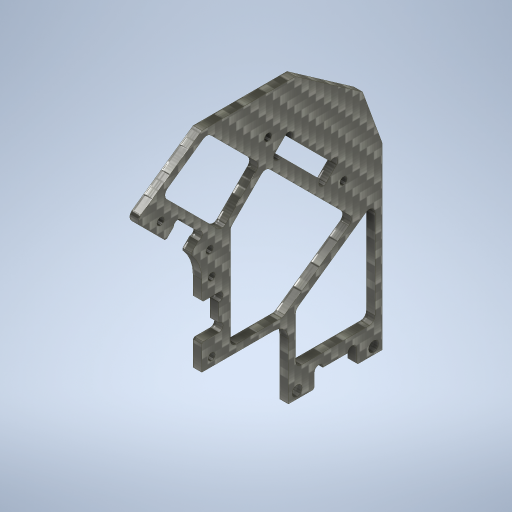
# Autodesk Inventor part: HeadSideFrame
Saved by Autodesk Inventor 2024.2 (Build 282272000, 272)
## iProperties
Created: 2024-01-28
Part Number: HeadSideFrame
Material: CFRP
Document SubType Name: Modeling
Designer: Masato Kubotera
Density: 1.43 g/cm^3
Appearance: Carbon Fiber 1
Mass: 10.5129 g
Surface Area: 73.9298 cm^2
Volume: 7.35165 cm^3
Vendor: meviy
Author: Masato Kubotera
Autodesk Inventor part; units mm, degrees
ref_plane "YZ Plane" through (0, 0, 0) normal (1, 0, 0) x (0, 1, 0)
ref_plane "XY Plane" through (0, 0, 0) normal (0, 0, 1) x (1, 0, 0)
ref_plane "Work Plane1" through (0, 30, 0) normal (0, 1, 0) x (-1, 0, 0)
sketch "Sketch1" plane through (0, 30, 0) normal (0, 1, 0) x (-1, 0, 0)
  line L0 (-16.25, -1.5) -> (16.25, -1.5)
  line L1 (-7.3, -1.5) -> (-7.3, 3.5)
  line L2 (7.3, 3.5) -> (7.3, -1.5)
  arc A0 (7.3, 3.5) -> (4.3, 3.5) centre (5.8, 3.5) ccw
  arc A1 (-4.3, 3.5) -> (-7.3, 3.5) centre (-5.8, 3.5) ccw
  line L3 (0, -1.5) -> (0, 3.5) construction
  line L4 (-13.25, 1) -> (13.25, 1) construction
  line L5 (-7.25, -1.5) -> (-7.25, 3.5) construction
  line L6 (7.25, -1.5) -> (7.25, 3.5) construction
  arc A2 (-47.5142, 62.9298) -> (-47.5142, 65.9298) centre (-47.5142, 64.4298) ccw
  line L7 (-62.6665, 77.5467) -> (-41.4533, 56.3335) construction
  line L8 (-33.1802, 64.6066) -> (-54.3934, 85.8198) construction
  line L9 (-53.8277, 65.1723) -> (-50.2922, 68.7078) construction
  arc A3 (-53.0702, 71.4858) -> (-56.0702, 71.4858) centre (-54.5702, 71.4858) ccw
  line L10 (-49.5851, 60.9296) -> (-46.0495, 64.4652) construction
  line L11 (-54.5348, 72.9505) -> (-49.5851, 60.9296) construction
  line L12 (-46.0495, 64.4652) -> (-54.5348, 72.9505) construction
  line L13 (-46.0495, 64.4652) -> (-58.0704, 69.4149) construction
  line L14 (-54.5348, 72.9505) -> (-58.0704, 69.4149) construction
  line L15 (-58.0704, 69.4149) -> (-49.5851, 60.9296) construction
  line L16 (-54.5702, 72.9858) -> (-58.7421, 68.8139)
  line L17 (-62.7373, 44.2419) -> (-46.0495, 60.9296) construction
  line L18 (-41.4533, 56.3335) -> (-33.1802, 64.6066) construction
  line L19 (-46.0142, 64.4298) -> (-54.5702, 72.9858)
  line L20 (-60.5452, 75.4253) -> (-43.5747, 58.4548) construction
  line L21 (-74.7581, 56.2627) -> (-62.7373, 44.2419) construction
  line L22 (-58.0704, 72.9505) -> (-74.7581, 56.2627) construction
  line L23 (-54.3934, 85.8198) -> (-62.6665, 77.5467) construction
  line L24 (-65, 54) -> (-119, 0) construction
  line L25 (0, 0) -> (-119, 0) construction
  line L26 (2.5776, 98) -> (57.5979, 98) construction
  line L27 (-7.3, 3.5) -> (7.3, 3.5)
  line L28 (-46.25, 98) -> (-46.25, 23) construction
  ellipse E0 centre (-46.25, 60.5) end of major axis (-46.25, 98) minor radius 30 (-46.25, 98) -> (-46.25, 23) ccw construction
  line L29 (-30, 98) -> (-30, 23) construction
  ellipse E1 centre (-13.75, 60.5) end of major axis (-13.75, 98) minor radius 30 (-13.75, 23) -> (-13.75, 98) ccw construction
  line L30 (-46.25, 98) -> (-13.75, 98) construction
  line L31 (-46.25, 23) -> (-13.75, 23) construction
  line L32 (-58.9896, 47.9896) -> (-71.0104, 60.0104) construction
  line L33 (-57.5883, 31.2154) -> (-87.7846, 61.4117) construction
  line L34 (-65, 54) -> (-57.5883, 31.2154) construction
  line L35 (-65, 54) -> (-87.7846, 61.4117) construction
  line L36 (-46.0142, 64.4298) -> (-50.1861, 60.2579)
  line L37 (-58.7421, 68.8139) -> (-69.2932, 79.365)
  line L38 (16.25, -1.5) -> (16.25, 60.5)
  line L39 (-16.25, -1.5) -> (-16.25, 23)
  line L40 (-20.8731, 76.0546) -> (-17.3376, 79.5901) construction
  line L41 (-17.3376, 79.5901) -> (0.3401, 61.9124) construction
  line L42 (0.3401, 61.9124) -> (-3.1954, 58.3769) construction
  line L43 (-3.1954, 58.3769) -> (-20.8731, 76.0546) construction
  line L44 (-20.8731, 76.0546) -> (0.3401, 61.9124) construction
  line L45 (-17.3376, 79.5901) -> (-3.1954, 58.3769) construction
  line L46 (-20.9438, 76.0546) -> (-17.3376, 79.6608)
  line L47 (-17.3376, 79.6608) -> (0.4108, 61.9124)
  line L48 (0.4108, 61.9124) -> (-3.1954, 58.3062)
  line L49 (-3.1954, 58.3062) -> (-20.9438, 76.0546)
  line L50 (-20.9438, 76.0546) -> (0.4108, 61.9124) construction
  line L51 (-17.3376, 79.6608) -> (-3.1954, 58.3062) construction
  arc A4 (-15.2163, 77.5395) -> (-17.3376, 79.6608) centre (-16.2769, 78.6001) ccw
  line L52 (-35.0152, 93.7322) -> (14.4822, 44.2348) construction
  line L53 (-8.4634, 70.7866) -> (-12.0696, 67.1804) construction
  arc A5 (-20.9438, 76.0546) -> (-18.8225, 73.9332) centre (-19.8832, 74.9939) ccw
  arc A6 (0.4108, 61.9124) -> (-1.7105, 64.0337) centre (-0.6499, 62.9731) ccw
  arc A7 (-5.3168, 60.4275) -> (-3.1954, 58.3062) centre (-4.2561, 59.3668) ccw
  line L54 (-46.25, 50.7553) -> (-46.25, 23)
  line L55 (-33.2475, 95.5) -> (-36.783, 91.9645) construction
  line L56 (-40.35, 32) -> (-46.25, 32) construction
  line L57 (-46.25, 44) -> (-40.35, 44) construction
  line L58 (-40.35, 44) -> (-40.35, 32) construction
  line L59 (-40.35, 32) -> (-46.25, 44) construction
  line L60 (-46.25, 32) -> (-40.35, 44) construction
  line L61 (-46.25, 44.05) -> (-40.35, 44.05)
  line L62 (-40.35, 44.05) -> (-40.35, 31.95)
  line L63 (-40.35, 31.95) -> (-46.25, 31.95)
  line L64 (-40.35, 38) -> (-46.25, 38) construction
  arc A8 (-40.35, 41.05) -> (-40.35, 44.05) centre (-40.35, 42.55) ccw
  line L65 (-42.85, 50) -> (-42.85, 26) construction
  line L66 (-46.25, 53) -> (-40.35, 53) construction
  arc A9 (-40.35, 31.95) -> (-40.35, 34.95) centre (-40.35, 33.45) ccw
  line L67 (-65.0707, 75.1425) -> (-60.8988, 79.3144) construction
  line L68 (-43.2211, 54.5657) -> (-39.6856, 58.1012) construction
  line L69 (-46.25, 60.5) -> (-76.25, 60.5) construction
  line L70 (-13.75, 60.5) -> (16.25, 60.5) construction
  line L71 (-11.75, 8) -> (11.75, 8)
  line L72 (-46.25, 95.5) -> (-13.75, 95.5)
  line L73 (-50.1861, 60.2579) -> (-46.25, 64.194)
  circle A10 centre (-42.85, 26) radius 2.4 construction
  circle A11 centre (-60.5452, 75.4253) radius 2.4 construction
  line L74 (-50.1861, 60.2579) -> (-50.1861, 60.2579)
  line L75 (4.9456, 44.5083) -> (-22.7522, 72.2061)
  line L76 (-25.5807, 72.2061) -> (-35.7642, 62.0226)
  line L77 (-36.35, 60.6084) -> (-36.35, 27.5)
  line L78 (-27.3484, 76.8023) -> (-43.1484, 92.6023)
  line L79 (-27.3484, 73.9739) -> (-37.9607, 63.3616)
  line L80 (-40.7891, 63.3616) -> (-58.4603, 81.0328)
  line L81 (-18.7392, 25.5) -> (-34.35, 25.5)
  line L82 (9.4147, 79.2799) -> (16.25, 60.5)
  line L83 (-13.75, 98) -> (-13.75, 23) construction
  line L84 (-13.75, 95.5) -> (9.4147, 79.2799)
  line L85 (16.25, 60.5) -> (9.4147, 41.7201)
  line L86 (9.4147, 41.7201) -> (-12.8972, 26.0972)
  line L87 (-46.25, 23) -> (-16.25, 23)
  line L88 (-13.75, 24.4589) -> (-13.75, 10)
  line L89 (13.75, 10) -> (13.75, 40.9137)
  line L90 (-46.25, 95.5) -> (-69.2932, 79.365)
  line L91 (9.4147, 41.7201) -> (10.6028, 42.552)
  line L92 (4.6786, 41.4558) -> (-17.5921, 25.8617)
  line L93 (-58.1932, 84.0853) -> (-45.7097, 92.8264)
  arc A12 (-43.1484, 92.6023) -> (-45.7097, 92.8264) centre (-44.5626, 91.1881) ccw
  arc A13 (-58.1932, 84.0853) -> (-58.4603, 81.0328) centre (-57.0461, 82.447) ccw
  arc A14 (-40.7891, 63.3616) -> (-37.9607, 63.3616) centre (-39.3749, 64.7758) ccw
  arc A15 (-27.3484, 73.9739) -> (-27.3484, 76.8023) centre (-28.7626, 75.3881) ccw
  arc A16 (-22.7522, 72.2061) -> (-25.5807, 72.2061) centre (-24.1665, 70.7919) ccw
  arc A17 (4.6786, 41.4558) -> (4.9456, 44.5083) centre (3.5314, 43.0941) ccw
  arc A18 (-18.7392, 25.5) -> (-17.5921, 25.8617) centre (-18.7392, 27.5) ccw
  arc A19 (-36.35, 27.5) -> (-34.35, 25.5) centre (-34.35, 27.5) ccw
  arc A20 (-35.7642, 62.0226) -> (-36.35, 60.6084) centre (-34.35, 60.6084) ccw
  arc A21 (13.75, 40.9137) -> (10.6028, 42.552) centre (11.75, 40.9137) ccw
  arc A22 (-12.8972, 26.0972) -> (-13.75, 24.4589) centre (-11.75, 24.4589) ccw
  arc A23 (-13.75, 10) -> (-11.75, 8) centre (-11.75, 10) ccw
  arc A24 (11.75, 8) -> (13.75, 10) centre (11.75, 10) ccw
  arc A25 (-46.25, 50.7553) -> (-50.1861, 60.2579) centre (-59.6887, 50.7553) ccw
  line L94 (12.7145, 42.467) -> (16.25, 46.0025) construction
  point P0 (-52.0599, 66.9401)
  point P1 (-47.5142, 65.9298)
  point P2 (-72.6865, 46.3135)
  point P3 (-76.1621, 57.6309)
  point P4 (-74.597, 48.2241)
  point P5 (-46.0142, 64.4298)
  point P6 (-46.0142, 64.4298)
  point P7 (-16.25, 34)
  point P8 (-10.2665, 68.9835)
  point P9 (-46.25, 56.3218)
  point P10 (-23.348, 82.065)
  point P11 (2.815, 55.902)
  point P12 (-1.7105, 64.0337)
  point P13 (-5.3168, 60.4275)
  point P14 (-18.8225, 73.9332)
  point P15 (-43.3, 38)
  point P16 (-40.35, 34.95)
  point P17 (-73.75, 60.5)
  point P18 (-13.75, 8)
  point P19 (13.75, 8)
  point P20 (16.25, 71.5)
  point P21 (-40.35, 45.95)
  point P22 (-47.0041, 71.6114)
  point P23 (6.631, 42.8229)
  point P24 (-24.1665, 73.6203)
  point P25 (-36.35, 61.4368)
  point P26 (-36.35, 25.5)
  point P27 (-25.9342, 75.3881)
  point P28 (-44.335, 93.7889)
  point P29 (-71.25, 60.5)
  point P30 (-39.3749, 61.9474)
  point P31 (-60.1457, 82.7182)
  point P32 (-13.75, 25.5)
  point P33 (13.75, 53.6313)
  point P34 (13.75, 44.7557)
  point P35 (-18.1086, 25.5)
  point P36 (-50.1861, 60.2579)
  dimension "d26" = 30
  dimension "d1" = 32.5
  dimension "d2" = 1.5
  dimension "d3" = 1.5
  dimension "d4" = 0.05
  dimension "d5" = 6
  dimension "d6" = 11.7
  dimension "d7" = 35.3
  dimension "d8" = 30
  dimension "d9" = 17
  dimension "d10" = 30
  dimension "d11" = 0.05
  dimension "d12" = 5
  dimension "d14" = 6
  dimension "d15" = 45
  dimension "d16" = 65
  dimension "d17" = 54
  dimension "d18" = 98
  dimension "d19" = 1.5
  dimension "d20" = 2.5
  dimension "d22" = 5
  dimension "d24" = 75
  dimension "d25" = 30
  dimension "d32" = 76.3675
  dimension "d34" = 10.8703
  dimension "d35" = 21.352
  dimension "d44" = 32.5
  dimension "d50" = 9
  dimension "d55" = 5
  dimension "d56" = 25
  dimension "d60" = 6
  dimension "d61" = 0.05
  dimension "d62" = 0.05
  dimension "d64" = 0.05
  dimension "d67" = 5.9
  dimension "d68" = 6
  dimension "d70" = 9
  dimension "d71" = 9
  dimension "d75" = 2.5
  dimension "d76" = 30
  dimension "d81" = 3
  dimension "d96" = 4.8
  dimension "d97" = 0.6
  dimension "d98" = 15
  dimension "d99" = 2.5
  dimension "d100" = 1
  dimension "d101" = 1
  dimension "d103" = 2.5
  dimension "d104" = 2.5
  dimension "d106" = 2.5
  dimension "d108" = 2.5
  dimension "d109" = 145
  dimension "d110" = 145
  dimension "d111" = 2.5
  dimension "d112" = 140
  dimension "d113" = 2
  dimension "d117" = 2.5
  dimension "d118" = 2.5
  dimension "d119" = 2.5
  dimension "d120" = 70
  dimension "d121" = 45
  dimension "d122" = 30
  constraints: 192 end point, 76 point on line, 49 point on circle, 28 tangent, 26 centre point, 24 midpoint, 23 symmetric about line, 16 equal radius, 16 parallel, 15 perpendicular, 14 horizontal, 12 collinear, 9 coincident, 8 vertical, 27 other
  measures "d1" distance of L0.start L0.end
  measures "d2" radius of A0
  measures "d3" distance from line of L0 L25.start
  measures "d4" distance between parallel lines of L2 L6
  measures "d5" distance from line of point (13.25, 1) L6
  measures "d6" distance of L7.end L8.start
  measures "d7" distance between parallel lines of L21 L8
  measures "d8" distance from line of L34.start L8
  measures "d9" distance between parallel lines of L17 L22
  measures "d10" distance of L8.start L8.end
  measures "d11" distance between parallel lines of L16 L14
  measures "d12" distance between parallel lines of L15 L12
  measures "d14" distance from line of L20.start L14
  measures "d15" angle of L24 L3
  measures "d16" horizontal distance of L25.start L34.start
  measures "d17" vertical distance of L25.start L34.start
  measures "d18" distance from line of L25.start L26
  measures "d19" radius of A3
  measures "d20" distance between parallel lines of L12 L7
  measures "d22" distance between parallel lines of L0 L27
  measures "d24" distance of L28.start L31.start
  measures "d25" distance from line of L25.start L29
  measures "d32" distance of L34.start L25.end
  measures "d34" distance from line of L33 L34.start
  measures "d35" distance of point (-72.686, 46.314) L33.end
  measures "d44" distance of L31.start L31.end
  measures "d50" distance from line of L0.end L6
  measures "d55" distance of L40.start L40.end
  measures "d56" distance of L40.end L41.end
  measures "d60" distance from line of L40 point (-23.348, 82.065)
  measures "d61" distance between parallel lines of L46 L40
  measures "d62" distance between parallel lines of L41 L47
  measures "d64" distance between parallel lines of L57 L61
  measures "d67" distance of L61.start L61.end
  measures "d68" distance from line of L57 L65.start
  measures "d70" distance between parallel lines of L57 L66
  measures "d71" distance between parallel lines of L67 L14
  measures "d75" distance of L69.end point (-73.75, 60.5)
  measures "d76" diameter of L66 L64
  measures "d81" distance edge to line of A0 L71
  measures "d96" diameter of A10
  measures "d97" distance edge to line of A10 L31
  measures "d98" distance between parallel lines of L31 L64
  measures "d99" distance between parallel lines of L62 L65
  measures "d100" distance edge to line of A10 L54
  measures "d101" distance edge to line of A11 L37
  measures "d103" distance edge to line of A9 L77
  measures "d104" distance edge to line of A7 L75
  measures "d106" distance of point (-73.75, 60.5) point (-71.25, 60.5)
  measures "d108" distance between parallel lines of L79 L76
  measures "d109" angle of L82 L84
  measures "d110" angle of L84 L72
  measures "d111" distance between parallel lines of L72 L30
  measures "d112" angle of L85 L82
  measures "d113" radius of A12
  measures "d117" distance between parallel lines of L86 L92
  measures "d118" distance between parallel lines of L90 L93
  measures "d119" distance edge to line of A2 L80
  measures "d120" distance between parallel lines of L94 L55
  measures "d121" angle of L29 L52
  measures "d122" distance between parallel lines of L68 L67
extrude "Extrusion1" add sketch "Sketch1" against normal blind 3 contours L39 L87 L54 L63 A9 L62 A8 L61 A25 L36 A2 L19 A3 L16 L37 L90 L72 L84 L82 L38 L0 L2 A0 L27 A1 L1
hole "Hole1" at (13.25, 30, 1) at (-13.25, 30, 1) direction (0, -1, 0) diameter 3.5 end through all
hole "Hole2" at (60.5452, 30, 75.4253) at (43.5747, 30, 58.4548) at (65, 30, 54) at (23.348, 30, 82.065) at (-2.815, 30, 55.902) at (42.85, 30, 50) at (42.85, 30, 26) at (73.75, 30, 60.5) direction (0, -1, 0) diameter 2.5 end through all
fillet "Fillet1" radius 5 1 edges at (16.25, 28.5, 23)
fillet "Fillet2" radius 2 1 edges at (69.2932, 28.5, 79.365)
chamfer "Chamfer1" distance 0.5 angle 45 6 edges at (58.7421, 28.5, 68.8139) (46.25, 28.5, 31.95) (46.25, 28.5, 44.05) (7.3, 28.5, -1.5) (-7.3, 28.5, -1.5) (50.1861, 28.5, 60.2579)
equation "\"d11\" = d28"
equation "\"d28\" = 0.05"
body "Solid1"
